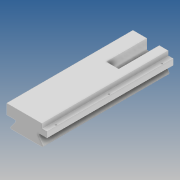
# Autodesk Inventor part: 3102_Dovetail Slider_V1
Saved by Autodesk Inventor 2020 (Build 240168000, 168)
## iProperties
Created: 2019-10-22
Part Number: 3102_Dovetail Slider_V1
Material: Generic
Document SubType Name: Modeling
Designer: RFLab
Density: 1 g/cm^3
Appearance: Default
Author: RFLab
Autodesk Inventor part; units mm, degrees
ref_plane "YZ Plane" through (0, 0, 0) normal (1, 0, 0) x (0, 1, 0)
ref_plane "XZ Plane" through (0, 0, 0) normal (0, 1, 0) x (-1, 0, 0)
ref_plane "XY Plane" through (0, 0, 0) normal (0, 0, 1) x (1, 0, 0)
sketch "Sketch1" plane through (0, 0, 0) normal (0, 0, 1) x (1, 0, 0)
  line L0 (-20, -10) -> (20, -10)
  line L1 (20, -10) -> (20, 10)
  line L2 (20, 10) -> (-20, 10)
  line L3 (-20, 10) -> (-20, -10)
  point P0 (0, 0)
  dimension "d0" = 40
  dimension "d1" = 20
  dimension "d2" = 10
  dimension "d3" = 20
  constraints: 8 end point, 2 parallel, 1 horizontal, 1 perpendicular
  measures "d0" distance of L1.end L2.end
  measures "d1" distance of L0.end L1.end
  measures "d2" distance from line of point (0, 0) L0
  measures "d3" distance from line of point (0, 0) L1
extrude "Extrusion1" add sketch "Sketch1" along normal blind 125
sketch "Sketch2" plane through (-20, 10, 0) normal (0, 1, 0) x (1, 0, 0)
  line L0 (40, 0) -> (0, 0) projected
  line L1 (13.9, 0) -> (26.1, 0)
  line L2 (26.1, 0) -> (26.1, -40.2)
  line L3 (26.1, -40.2) -> (13.9, -40.2)
  line L4 (13.9, -40.2) -> (13.9, 0)
  point P0 (20, 0)
  point P1 (26.1, 0)
  dimension "d6" = 40.2
  dimension "d7" = 12.2
  dimension "d8" = 13.9
  constraints: 8 end point, 2 parallel, 1 horizontal, 1 perpendicular, 1 point on line
  measures "d6" distance of L3.end L1.start
  measures "d7" distance of L2.end L3.end
  measures "d8" distance of L0.end L1.start
extrude "Extrusion2" cut sketch "Sketch2" against normal blind 10
sketch "Sketch3" plane through (-20, 10, 125) normal (0, 1, 0) x (1, 0, 0)
  line L0 (40, 125) -> (40, 0) projected
  line L1 (40, 125) -> (26.1, 125) projected
  line L2 (40, 0) -> (35, 0)
  line L3 (35, 0) -> (35, 125)
  line L4 (35, 125) -> (40, 125)
  line L5 (40, 125) -> (40, 0)
  point P0 (20, 125)
  dimension "d11" = 5
  constraints: 8 end point, 2 parallel, 1 horizontal, 1 perpendicular, 1 point on line
  measures "d11" distance of L0.end L2.end
extrude "Extrusion3" cut sketch "Sketch3" against normal blind 4.3
sketch "Sketch4" plane through (-20, 0, 0) normal (0, 1, 0) x (1, 0, 0)
  circle A0 centre (20, -10.1) radius 1.25
  line L0 (13.9, 0) -> (26.1, 0) projected
  line L1 (13.9, -40.2) -> (13.9, 0) projected
  circle A1 centre (20, -30.1) radius 1.25
  point P0 (20, 0)
  dimension "d14" = 2.5
  dimension "d15" = 10.1
  dimension "d16" = 6.1
  dimension "d35" = 20
  dimension "d36" = 6.1
  constraints: 2 centre point, 1 equal radius
  measures "d14" diameter of A0
  measures "d15" distance from line of L0 A0.centre
  measures "d16" distance from line of L1 A0.centre
  measures "d35" distance of A1.centre A0.centre
  measures "d36" distance from line of L1 A1.centre
extrude "Extrusion4" cut sketch "Sketch4" against normal through all
sketch "Sketch5" plane through (0, 0, 125) normal (0, 0, 1) x (1, 0, 0)
  line L0 (-20, 10) -> (-20, -10) projected
  line L1 (20, -10) -> (20, 5.7) projected
  line L2 (-20, 0) -> (-10, 0)
  line L3 (-10, 0) -> (-20, -10)
  line L4 (-20, 0) -> (-20, -10)
  line L5 (20, 0) -> (20, -10)
  line L6 (20, 0) -> (10, 0)
  line L7 (10, 0) -> (20, -10)
  line L8 (-20, -10) -> (-17, -10)
  line L9 (-20, -10) -> (20, -10) projected
  line L10 (-10, 0) -> (-17, -10)
  line L11 (10, 0) -> (17, -10)
  line L12 (17, -10) -> (20, -10)
  point P0 (0, 0)
  dimension "d19" = 10
  dimension "d21" = 10
  dimension "d24" = 3
  dimension "d25" = 3
  constraints: 20 end point, 3 collinear, 3 point on line, 2 horizontal, 1 midpoint
  measures "d19" distance of L2.start L2.end
  measures "d21" distance of L5.start L6.end
  measures "d24" distance of L0.end L8.end
  measures "d25" distance of L11.end L1.start
extrude "Extrusion5" cut sketch "Sketch5" against normal through all
fillet "Fillet1" radius 1 4 edges at (17, -10, 62.5) (10, 0, 62.5) (-17, -10, 62.5) (-10, 0, 62.5)
sketch "Sketch6" plane through (-20, 5.7, 125) normal (0, 1, 0) x (1, 0, 0)
  circle A0 centre (38.734, 10) radius 0.81
  circle A1 centre (38.734, 115) radius 0.81
  line L0 (40, 0) -> (35, 0) projected
  line L1 (35, 125) -> (40, 125) projected
  line L2 (35, 0) -> (35, 125) projected
  circle A2 centre (38.734, 62.5) radius 0.81
  point P0 (20, 125)
  dimension "d27" = 1.62
  dimension "d28" = 1.62
  dimension "d29" = 10
  dimension "d30" = 10
  dimension "d31" = 3.734
  dimension "d32" = 3.734
  dimension "d37" = 3.734
  dimension "d38" = 1.62
  dimension "d39" = 52.5
  dimension "d40" = 52.5
  constraints: 3 centre point
  measures "d27" diameter of A0
  measures "d28" diameter of A1
  measures "d29" distance from line of L0 A0.centre
  measures "d30" distance from line of L1 A1.centre
  measures "d31" distance from line of L2 A0.centre
  measures "d32" distance from line of L2 A1.centre
  measures "d37" distance from line of L2 A2.centre
  measures "d38" diameter of A2
  measures "d39" distance of A0.centre A2.centre
  measures "d40" distance of A1.centre A2.centre
extrude "Extrusion6" cut sketch "Sketch6" against normal up to surface (5.7 mm away)
equation "\"d2\" = 0.5 * d1"
equation "\"d3\" = 0.5 * d0"
equation "\"d32\" = d31"
equation "\"d37\" = d31"
equation "\"d38\" = d27"
body "Solid1"
